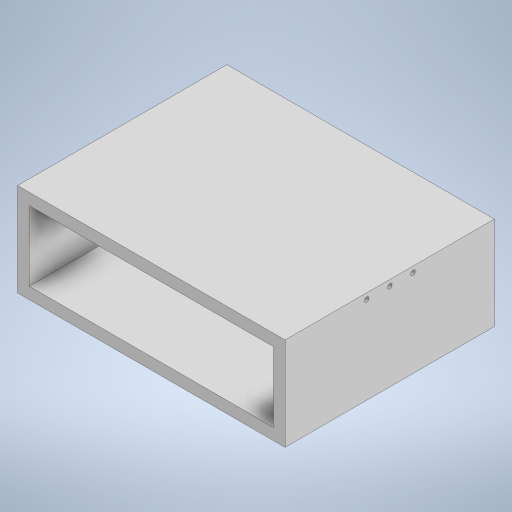
# Autodesk Inventor part: BatteryBoxV2-Bottom
Saved by Autodesk Inventor 2024 (Build 280153000, 153)
## iProperties
Created: 2025-03-26
Part Number: BatteryBoxV2-Bottom
Material: Generic
Document SubType Name: Modeling
Designer: v
Density: 1 g/cm^3
Appearance: Default
Author: v
Autodesk Inventor part; units mm, degrees
ref_plane "YZ Plane" through (0, 0, 0) normal (1, 0, 0) x (0, 1, 0)
ref_plane "XZ Plane" through (0, 0, 0) normal (0, 1, 0) x (-1, 0, 0)
ref_plane "XY Plane" through (0, 0, 0) normal (0, 0, 1) x (1, 0, 0)
sketch "BottomBoxFrame" plane through (0, 0, 0) normal (0, 0, 1) x (1, 0, 0)
  line L0 (0, 0) -> (292.1, 0)
  line L1 (292.1, 0) -> (292.1, 101.6)
  line L2 (292.1, 101.6) -> (0, 101.6)
  line L3 (0, 101.6) -> (0, 0)
  dimension "d0" = 101.6
  dimension "d1" = 292.1
  constraints: 8 end point, 2 parallel, 1 horizontal, 1 perpendicular
  measures "d0" distance of L0.end L1.end
  measures "d1" distance of L0.start L0.end
extrude "BottomBoxWidth" add sketch "BottomBoxFrame" against normal blind 228.6
sketch "TrayShape" plane through (0, 0, 0) normal (0, 0, 1) x (1, 0, 0)
  line L0 (12.7, 12.7) -> (279.4, 12.7)
  line L1 (279.4, 12.7) -> (279.4, 88.9)
  line L2 (279.4, 88.9) -> (12.7, 88.9)
  line L3 (12.7, 88.9) -> (12.7, 12.7)
  line L4 (0, 0) -> (292.1, 0) projected
  line L5 (0, 101.6) -> (0, 0) projected
  line L6 (292.1, 0) -> (292.1, 101.6) projected
  line L7 (292.1, 101.6) -> (0, 101.6) projected
  dimension "d5" = 12.7
  dimension "d6" = 12.7
  dimension "d7" = 12.7
  dimension "d10" = 12.7
  constraints: 8 end point, 2 parallel, 1 horizontal, 1 perpendicular
  measures "d5" distance between parallel lines of L4 L0
  measures "d6" distance between parallel lines of L5 L3
  measures "d7" distance between parallel lines of L6 L1
  measures "d10" distance between parallel lines of L7 L2
extrude "TrayCut" cut sketch "TrayShape" against normal blind 215.9 contours L3 L2 L1 L0
sketch "RightHoleGeo" plane through (292.1, 0, 0) normal (1, 0, 0) x (0, 0, -1)
  line L0 (0, 101.6) -> (228.6, 101.6) projected
  line L1 (0, 0) -> (0, 101.6) projected
  point P0 (88.9, 95.25)
  point P1 (114.3, 95.25)
  point P2 (139.7, 95.25)
  dimension "d18" = 6.35
  dimension "d19" = 88.9
  dimension "d22" = 25.4
  constraints: 1 horizontal, 2 other
  measures "d18" distance from line of L0 point (88.9, 95.25)
  measures "d19" distance from line of L1 point (88.9, 95.25)
  measures "d22" distance of point (88.9, 95.25) point (114.3, 95.25)
hole "RightPlateHoles" at (292.1, 95.25, -88.9) at (292.1, 95.25, -114.3) at (292.1, 95.25, -139.7) direction (-1, 0, 0) diameter 5.1054 depth 50.8 tip angle 118 clearance for "Flat Head Machine Screw (82)" size "#10" standard "Ansi Unified Screw Threads"
sketch "LeftHoleGeo" plane through (0, 0, 0) normal (-1, 0, 0) x (0, 0, 1)
  line L0 (0, 101.6) -> (-228.6, 101.6) projected
  line L1 (-228.6, 0) -> (-228.6, 101.6) projected
  point P0 (0, 0)
  point P1 (-139.7, 95.25)
  point P2 (-114.3, 95.25)
  point P3 (-88.9, 95.25)
  dimension "d34" = 6.35
  dimension "d35" = 88.9
  dimension "d38" = 25.4
  constraints: 1 horizontal, 2 other
  measures "d34" distance from line of L0 point (-139.7, 95.25)
  measures "d35" distance from line of L1 point (-139.7, 95.25)
  measures "d38" distance of point (-139.7, 95.25) point (-114.3, 95.25)
hole "LeftPlateHoles" at (0, 95.25, -139.7) at (0, 95.25, -114.3) at (0, 95.25, -88.9) direction (1, 0, 0) diameter 5.1054 depth 50.8 tip angle 118 clearance for "Flat Head Machine Screw (82)" size "#10" standard "Ansi Unified Screw Threads"
equation "\"d6\" = d5"
equation "\"d7\" = d6"
equation "\"d10\" = d5"
body "Solid1"
